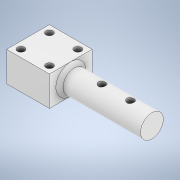
# Autodesk Inventor part: RodConnector
Saved by Autodesk Inventor 2022.1 (Build 261234020, 234B)
## iProperties
Created: 2021-11-12
Part Number: RodConnector
Material: ABS Plastic
Document SubType Name: Modeling
Designer: Alexander
Density: 1.06 g/cm^3
Appearance: Smooth - White
Author: Alexander
## iProperties of the stored document RodConnector_3DPrint.ipt
Created: 2021-11-12
Part Number: RodConnector_3DPrint
Material: Generic
Document SubType Name: Modeling
Designer: Alexander
Density: 1 g/cm^3
Appearance: Default
Author: Alexander
Autodesk Inventor part; units mm, degrees
ref_plane "YZ Plane" through (0, 0, 0) normal (1, 0, 0) x (0, 1, 0)
ref_plane "XZ Plane" through (0, 0, 0) normal (0, 1, 0) x (-1, 0, 0)
ref_plane "XY Plane" through (0, 0, 0) normal (0, 0, 1) x (1, 0, 0)
sketch "Sketch1" plane through (0, 0, 0) normal (0, 1, 0) x (-1, 0, 0)
  line L0 (-15, -15) -> (15, -15)
  line L1 (15, -15) -> (15, 15)
  line L2 (15, 15) -> (-15, 15)
  line L3 (-15, 15) -> (-15, -15)
  line L4 (-15, -15) -> (15, 15) construction
  line L5 (15, -15) -> (-15, 15) construction
  point P0 (0, 0)
  dimension "d0" = 30
  dimension "d1" = 30
  constraints: 12 end point, 2 midpoint, 2 parallel, 1 horizontal, 1 perpendicular
  measures "d0" distance of L2.end L1.end
  measures "d1" distance of L1.end L0.end
extrude "Extrusion1" add sketch "Sketch1" along normal blind 21
sketch "Sketch2" plane through (15, 0, 15) normal (1, 0, 0) x (0, 0, -1)
  circle A0 centre (15, 10.5) radius 8
  line L0 (0, 21) -> (30, 21) projected
  point P0 (15, 0)
  point P1 (15, 21)
  dimension "d4" = 16
  dimension "d29" = 10.5
  constraints: 1 centre point, 1 midpoint
  measures "d4" diameter of A0
  measures "d29" distance of point (15, 21) A0.centre
extrude "Extrusion2" add sketch "Sketch2" along normal blind 57
sketch "Sketch3" plane through (0, 21, 0) normal (0, 1, 0) x (1, 0, 0)
  circle A0 centre (37, 0) radius 2.5
  circle A1 centre (57, 0) radius 2.5
  line L0 (15, -15) -> (15, 15) projected
  line L1 (72, -8) -> (72, 8) projected
  circle A2 centre (10, -10) radius 2.5
  line L2 (1.0234, -33.583) -> (-6.5136, -33.583)
  line L3 (-6.5136, -33.583) -> (-6.5136, -27.1544)
  circle A3 centre (-10, -10) radius 2.5
  circle A4 centre (10, 10) radius 2.5
  circle A5 centre (-10, 10) radius 2.5
  line L4 (-15, -15) -> (15, -15) projected
  line L5 (-15, 15) -> (-15, -15) projected
  point P0 (0, 0)
  point P1 (15, 0)
  point P2 (72, 0)
  dimension "d7" = 5
  dimension "d8" = 5
  dimension "d9" = 22
  dimension "d10" = 20
  dimension "d12" = 5
  dimension "d15" = 20
  dimension "d18" = 20
  dimension "d21" = 5
  dimension "d22" = 5
  dimension "d28" = 15
  constraints: 6 centre point, 4 end point, 2 horizontal, 1 midpoint, 1 perpendicular, 1 vertical, 6 other
  measures "d7" diameter of A0
  measures "d8" diameter of A1
  measures "d9" distance from line of L0 A0.centre
  measures "d10" distance of A1.centre A0.centre
  measures "d12" diameter of A2
  measures "d15" distance of A2.centre A3.centre
  measures "d18" distance of A2.centre A4.centre
  measures "d21" distance from line of L4 A3.centre
  measures "d22" distance from line of L5 A3.centre
  measures "d28" distance of point (72, 0) A1.centre
chamfer "Chamfer1" distance 2.5 angle 45 1 edges at (15, 10.5, 8)
extrude "Extrusion4" cut sketch "Sketch3" against normal through all contours A2 | A3 | A4 | A5
extrude "Extrusion5" cut sketch "Sketch3" against normal through all contours A0 | A1
body "Solid1"
